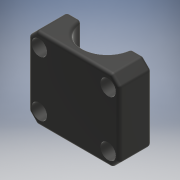
# Autodesk Inventor part: hotend_holder_pulley
Saved by Autodesk Inventor 2018 (Build 220112000, 112)
## iProperties
Created: 2018-07-15
Part Number: hotend_holder_pulley
Material: ABS Plastic
Document SubType Name: Modeling
Designer: Z. Deniz
Density: 1.06 g/cm^3
Appearance: Smooth - White
Author: Z. Deniz
Autodesk Inventor part; units mm, degrees
ref_plane "YZ Plane" through (0, 0, 0) normal (1, 0, 0) x (0, 1, 0)
ref_plane "XZ Plane" through (0, 0, 0) normal (0, 1, 0) x (-1, 0, 0)
ref_plane "XY Plane" through (0, 0, 0) normal (0, 0, 1) x (1, 0, 0)
sketch "Sketch1" plane through (0, 0, 0) normal (0, 1, 0) x (-1, 0, 0)
  line L0 (0, 0) -> (-28, 0)
  line L1 (-28, 0) -> (-28, -25)
  line L2 (-28, -25) -> (0, -25)
  line L3 (0, -25) -> (0, 0)
  line L4 (-24.8835, -25) -> (-24.8835, 0) construction
  line L5 (0, -1.9376) -> (-28, -1.9376) construction
  line L6 (-2.7003, -25) -> (-2.7003, 0) construction
  line L7 (0, -22.688) -> (-28, -22.688) construction
  line L8 (-34, -12.5) -> (0, -12.5) construction
  circle A0 centre (-34, -12.5) radius 6
  circle A1 centre (-34, -12.5) radius 9
  dimension "d0" = 28
  dimension "d1" = 25
  dimension "d31" = 12
  dimension "d32" = 12.5
  dimension "d33" = 18
  constraints: 18 end point, 8 point on line, 5 perpendicular, 2 centre point, 2 coincident, 2 parallel, 1 horizontal, 1 midpoint, 1 tangent
  measures "d0" distance of L2.end L1.end
  measures "d1" distance of L1.end L0.end
  measures "d31" diameter of A0
  measures "d32" distance between parallel lines of L0 L8
  measures "d33" diameter of A1
extrude "Extrusion1" add sketch "Sketch1" along normal blind 10 contours L3 L2 L1 A1 L0 | A1 L1 picked at (-27.5773, -8.4946)
sketch "Sketch2" plane through (0, 0, 0) normal (0, 0, 1) x (1, 0, 0)
  line L0 (0, 0) -> (28, 0) projected
  line L1 (28, 0) -> (28, 10) projected
  line L2 (0, 10) -> (28, 10) projected
  line L3 (0, 0) -> (0, 10) projected
  line L4 (0, 0) -> (0, 10) construction
  line L5 (0, 2.75) -> (28, 2.75) construction
  line L6 (28, 0) -> (28, 10) construction
  circle A0 centre (14, 10.325) radius 7.575
  line L7 (0, 10) -> (28, 10) construction
  line L8 (14, 10) -> (14, 2.75) construction
  dimension "d4" = 7.25
  dimension "d5" = 15.15
  constraints: 4 end point, 3 point on line, 2 midpoint, 1 centre point, 1 perpendicular, 1 tangent
  measures "d4" distance between parallel lines of L5 L2
  measures "d5" diameter of A0
extrude "Extrusion2" cut sketch "Sketch2" against normal through all contours A0 L2 | L2 A0
sketch "Sketch3" plane through (0, 10, 0) normal (0, 1, 0) x (1, 0, 0)
  line L0 (6.432, 0) -> (6.432, 25) projected
  line L1 (6.432, 25) -> (0, 25) projected
  line L2 (0, 25) -> (0, 0) projected
  line L3 (0, 0) -> (6.432, 0) projected
  line L4 (21.568, 25) -> (21.568, 0) projected
  line L5 (21.568, 0) -> (28, 0) projected
  line L6 (28, 0) -> (28, 25) projected
  line L7 (28, 25) -> (21.568, 25) projected
  line L8 (0, 21) -> (28, 21) construction
  line L9 (28, 0) -> (28, 25) construction
  line L10 (6.432, 25) -> (0, 25) construction
  line L11 (3.432, 25) -> (3.432, 0) construction
  line L12 (0, 0) -> (28, 0) construction
  line L13 (28, 25) -> (0, 25) construction
  line L14 (24.568, 25) -> (24.568, 0) construction
  line L15 (0, 25) -> (0, 0) construction
  line L16 (0, 4) -> (28, 4) construction
  circle A0 centre (3.432, 21) radius 1.625
  circle A1 centre (24.568, 21) radius 1.625
  circle A2 centre (3.432, 4) radius 1.625
  circle A3 centre (24.568, 4) radius 1.625
  dimension "d8" = 4
  dimension "d9" = 4
  dimension "d10" = 3
  dimension "d11" = 3
  dimension "d12" = 3.25
  dimension "d13" = 3.25
  dimension "d14" = 3.25
  dimension "d15" = 3.25
  constraints: 16 point on line, 8 end point, 4 centre point, 3 perpendicular, 1 parallel
  measures "d8" distance between parallel lines of L8 L1
  measures "d9" distance between parallel lines of L3 L16
  measures "d10" distance between parallel lines of L11 L0
  measures "d11" distance between parallel lines of L4 L14
  measures "d12" diameter of A0
  measures "d13" diameter of A1
  measures "d14" diameter of A2
  measures "d15" diameter of A3
extrude "Extrusion3" cut sketch "Sketch3" against normal through all contours A0 | A1 | A2 | A3
chamfer "Chamfer1" distance 2.5 angle 45 4 edges at (0, 5, 0) (28, 5, 0) (28, 5, -25) (0, 5, -25)
fillet "Fillet1" radius 1 30 edges at (14, 0, -25) (2.5, 5, -25) (0, 5, -22.5) (1.25, 0, -23.75) (14, 2.75, -25) (14, 2.75, 0) (6.432, 10, -12.5) (21.568, 10, -12.5) (0, 10, -12.5) (1.25, 10, -1.25) (4.466, 10, 0) (4.466, 10, -25) (1.25, 10, -23.75) (23.534, 10, -25) (25.5, 5, -25) (28, 5, -22.5) (26.75, 0, -23.75) (26.75, 10, -23.75) (28, 10, -12.5) (26.75, 10, -1.25) (23.534, 10, 0) (28, 0, -12.5) (28, 5, -2.5) (26.75, 0, -1.25) (14, 0, 0) (1.25, 0, -1.25) (0, 0, -12.5) (25.5, 5, 0) (2.5, 5, 0) (0, 5, -2.5)
sketch "Sketch5" plane through (0, 0, 0) normal (0, -1, 0) x (1, 0, 0)
  circle A0 centre (3.432, -4) radius 1.625 projected
  circle A1 centre (3.432, -4) radius 2.375
  circle A2 centre (3.432, -21) radius 1.625 projected
  circle A3 centre (24.568, -21) radius 1.625 projected
  circle A4 centre (24.568, -4) radius 1.625 projected
  circle A5 centre (3.432, -21) radius 2.375
  circle A6 centre (24.568, -21) radius 2.375
  circle A7 centre (24.568, -4) radius 2.375
  point P0 (0, 0)
  dimension "d22" = 4.75
  dimension "d23" = 4.75
  dimension "d24" = 4.75
  dimension "d25" = 4.75
  constraints: 4 centre point, 4 coincident
  measures "d22" diameter of A1
  measures "d23" diameter of A5
  measures "d24" diameter of A6
  measures "d25" diameter of A7
extrude "Extrusion4" cut sketch "Sketch5" against normal blind 5
equation "\"d9\" = d8"
equation "\"d11\" = d10"
equation "\"d13\" = d12"
equation "\"d14\" = d12"
equation "\"d15\" = d12"
body "Solid1"
